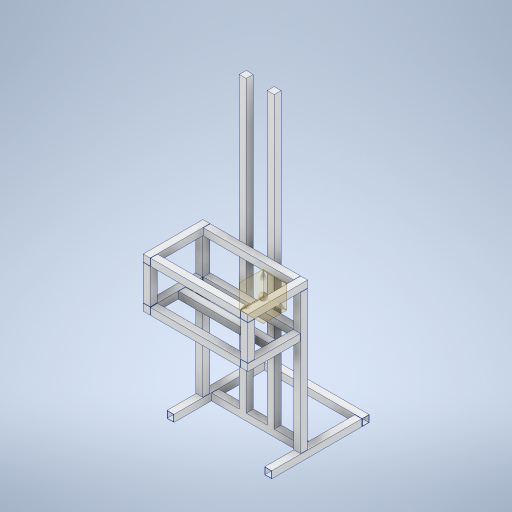
# Autodesk Inventor part: Новый каркас
Saved by Autodesk Inventor 2023 (Build 270158000, 158)
## iProperties
Created: 2022-04-27
Part Number: Новый каркас
Material: Алюминий 6061
Document SubType Name: Modeling
Designer: avkap
Density: 2.7 g/cm^3
Appearance: Алюминий — плоский
Mass: 63771.5 g
Surface Area: 27844 cm^2
Volume: 23619.1 cm^3
Author: avkap
Autodesk Inventor part; units mm, degrees
ref_plane "YZ Plane" through (0, 0, 0) normal (1, 0, 0) x (0, 1, 0)
ref_plane "XZ Plane" through (0, 0, 0) normal (0, 1, 0) x (-1, 0, 0)
ref_plane "XY Plane" through (0, 0, 0) normal (0, 0, 1) x (1, 0, 0)
sketch "Эскиз1" plane through (0, 0, 0) normal (0, 1, 0) x (-1, 0, 0)
  line L0 (-600, 0) -> (-600, -300)
  line L1 (-600, -300) -> (0, -300)
  line L2 (0, -300) -> (0, -42)
  line L3 (-600, 0) -> (-600, -40)
  line L4 (0, -300) -> (0, -260)
  line L5 (0, -260) -> (-600, -260)
  line L6 (-600, -40) -> (-600, -42)
  line L7 (-600, -42) -> (-560, -42)
  line L8 (-560, -42) -> (-560, -208)
  line L9 (0, -42) -> (-40, -42)
  line L10 (-40, -42) -> (-40, -258)
  line L11 (-40, -258) -> (0, -258)
  line L12 (-560, -208) -> (-560, -258)
  line L13 (-560, -258) -> (-600, -258)
  point P0 (0, 0)
  point P1 (-600, -208)
  dimension "d0" = 600
  dimension "d1" = 300
  dimension "d3" = 40
  dimension "d4" = 2
  dimension "d5" = 40
  dimension "d7" = 40
  dimension "d69" = 216
  constraints: 28 end point, 10 point on line, 4 perpendicular, 2 parallel
  measures "d0" distance of L1.end L0.end
  measures "d1" distance of L0.end L0.start
  measures "d3" distance of L1.end L4.end
  measures "d4" distance of L3.end L6.end
  measures "d5" distance of L6.end L7.end
  measures "d7" distance of L2.end L9.end
  measures "d69" distance of L9.end L10.end
ref_plane "РабПлоскость2" through (0, 860, 0) normal (0, 1, 0) x (1, 0, 0)
ref_plane "РабПлоскость6" through (0, 0, 0) normal (0, -1, 0) x (1, 0, 0)
sketch "Эскиз5" plane through (0, 0, 0) normal (0, -1, 0) x (1, 0, 0)
  line L0 (0, 0) -> (40, 0) projected
  line L1 (0, 0) -> (300, 0)
  line L2 (300, 0) -> (300, 2)
  line L3 (300, 2) -> (280, 2)
  line L4 (320, 2) -> (300, 2)
  line L5 (300, 2) -> (200, 2)
  line L6 (200, 2) -> (200, 4)
  line L7 (200, 4) -> (400, 4)
  line L8 (200, 4) -> (240, 4)
  line L9 (240, 4) -> (240, 44)
  line L10 (240, 44) -> (200, 44)
  line L11 (200, 44) -> (200, 4)
  line L12 (400, 4) -> (360, 4)
  line L13 (360, 4) -> (360, 44)
  line L14 (360, 44) -> (400, 44)
  line L15 (400, 44) -> (400, 4)
  dimension "d19" = 300
  dimension "d20" = 2
  dimension "d146" = 100
  dimension "d147" = 2
  dimension "d148" = 200
  dimension "d149" = 40
  dimension "d150" = 40
  dimension "d151" = 40
  dimension "d152" = 40
  constraints: 30 end point, 4 parallel, 4 perpendicular, 2 collinear, 2 horizontal, 2 point on line, 2 vertical
  measures "d19" distance of L0.start L1.end
  measures "d20" distance of L1.end L2.end
  measures "d146" distance of L2.end L5.end
  measures "d147" distance of L5.end L6.end
  measures "d148" distance of L6.end L7.end
  measures "d149" distance of L10.end L9.end
  measures "d150" distance of L9.end L8.end
  measures "d151" distance of L13.end L14.end
  measures "d152" distance of L12.end L13.end
extrude "Выдавливание10" add sketch "Эскиз1" along normal blind 40
extrude "Выдавливание20" add sketch "Эскиз5" against normal blind 1700
ref_plane "РабПлоскость16" through (200, 900, 44) normal (0, 0, 1) x (1, 0, 0)
sketch "Эскиз19" plane through (200, 900, 44) normal (0, 0, 1) x (1, 0, 0)
  line L0 (0, -900) -> (0, 800) projected
  line L1 (0, 800) -> (200, 800)
  line L2 (200, 800) -> (200, 600)
  line L3 (200, 600) -> (0, 600)
  line L4 (0, 600) -> (0, 800)
  line L5 (100, 600) -> (100, 800)
  line L6 (100, 600) -> (100, 700)
  line L7 (100, 700) -> (100, 692.5)
  line L8 (100, 692.5) -> (100, 709.5)
  circle A0 centre (100, 709.5) radius 2
  circle A1 centre (100, 692.5) radius 2
  line L9 (40, 800) -> (0, 800) projected
  line L10 (20, 800) -> (20, 600)
  line L11 (160, 800) -> (200, 800) projected
  line L12 (180, 800) -> (180, 600)
  line L13 (180, 600) -> (180, 620)
  line L14 (180, 620) -> (20, 620)
  line L15 (40, 800) -> (20, 800)
  line L16 (20, 800) -> (20, 780)
  line L17 (20, 780) -> (40, 780)
  line L18 (40, 780) -> (40, 800)
  line L19 (40, 780) -> (200, 780)
  circle A2 centre (20, 780) radius 3
  circle A3 centre (20, 620) radius 3
  circle A4 centre (180, 780) radius 3
  circle A5 centre (180, 620) radius 3
  point P0 (-200, -900)
  dimension "d156" = 200
  dimension "d157" = 200
  dimension "d266" = 100
  dimension "d267" = 7.5
  dimension "d268" = 17
  dimension "d269" = 4
  dimension "d270" = 4
  dimension "d271" = 20
  dimension "d272" = 20
  dimension "d273" = 20
  dimension "d274" = 6
  dimension "d275" = 6
  dimension "d276" = 6
  dimension "d277" = 6
  constraints: 34 end point, 9 point on line, 6 centre point, 5 coincident, 5 midpoint, 4 parallel, 3 horizontal, 3 perpendicular
  measures "d156" distance of L2.end L3.end
  measures "d157" distance of L1.end L2.end
  measures "d266" distance of L5.start L6.end
  measures "d267" distance of L6.end L7.end
  measures "d268" distance of L7.end L8.end
  measures "d269" diameter of A0
  measures "d270" diameter of A1
  measures "d271" distance of L12.end L13.end
  measures "d272" distance of L17.end L16.end
  measures "d273" distance of L16.end L15.end
  measures "d274" diameter of A2
  measures "d275" diameter of A3
  measures "d276" diameter of A4
  measures "d277" diameter of A5
extrude "Выдавливание21" [suppressed]
sketch "Эскиз23" plane through (560, 0, -42) normal (0, 0, 1) x (1, 0, 0)
  line L0 (-520, 0) -> (-520, 40) projected
  line L1 (-520, 0) -> (-560, 0)
  line L2 (-560, 0) -> (-560, 40)
  line L3 (-560, 40) -> (-520, 40)
  line L4 (-520, 40) -> (-520, 0)
  line L5 (40, 0) -> (40, 40) projected
  line L6 (40, 0) -> (0, 0)
  line L7 (0, 0) -> (0, 40)
  line L8 (0, 40) -> (40, 40)
  line L9 (40, 40) -> (40, 0)
  constraints: 16 end point, 4 parallel, 2 horizontal, 2 perpendicular
extrude "Выдавливание25" add sketch "Эскиз23" along normal blind 300
ref_plane "РабПлоскость12" through (42, 0, -258) normal (1, 0, 0) x (0, 0, -1)
sketch "Эскиз26" plane through (42, 0, -258) normal (1, 0, 0) x (0, 0, -1)
  line L0 (-302, 40) -> (-262, 40)
  line L1 (-262, 40) -> (-262, 0)
  line L2 (-262, 0) -> (-302, 0)
  line L3 (-302, 0) -> (-302, 40)
  line L4 (-262, 0) -> (0, 0)
  line L5 (0, 0) -> (0, 40) projected
  line L6 (0, 0) -> (0, 40)
  line L7 (-302, 0) -> (-302, 1700) projected
  point P0 (-258, 0)
  point P1 (-302, 1500)
  dimension "d189" = 40
  dimension "d302" = 262
  constraints: 12 end point, 2 horizontal, 2 parallel, 2 perpendicular
  measures "d189" distance of L1.end L2.end
  measures "d302" distance of L1.end L4.end
extrude "Выдавливание26" add sketch "Эскиз26" along normal blind 516
ref_plane "РабПлоскость22" through (0, 600, 0) normal (0, -1, 0) x (1, 0, 0)
ref_plane "РабПлоскость15" through (0, 42, 0) normal (0, 1, 0) x (1, 0, 0)
sketch "Эскиз30" plane through (0, 42, 0) normal (0, 1, 0) x (1, 0, 0)
  line L0 (40, 258) -> (40, -258) projected
  line L1 (40, -52.0658) -> (0, -52.0658)
  line L2 (0, -52.0658) -> (0, -92.0658)
  line L3 (0, -92.0658) -> (40, -92.0658)
  line L4 (40, -92.0658) -> (40, -52.0658)
  line L5 (560, 258) -> (560, -258) projected
  line L6 (560, -52.0658) -> (600, -52.0658)
  line L7 (600, -52.0658) -> (600, -92.0658)
  line L8 (600, -92.0658) -> (560, -92.0658)
  line L9 (560, -92.0658) -> (560, -52.0658)
  point P0 (0, 0)
  dimension "d217" = 40
  dimension "d218" = 40
  constraints: 16 end point, 4 parallel, 4 point on line, 2 horizontal, 2 perpendicular
  measures "d217" distance of L3.end L2.end
  measures "d218" distance of L2.end L1.end
extrude "Выдавливание28" add sketch "Эскиз30" along normal blind 800
ref_plane "РабПлоскость18" through (0, 844, 0) normal (0, 1, 0) x (1, 0, 0)
ref_plane "РабПлоскость21" through (42, 600, 294) normal (1, 0, 0) x (0, 0, -1)
sketch "Эскиз40" plane through (42, 600, 294) normal (1, 0, 0) x (0, 0, -1)
  line L0 (200, 40) -> (200, 0)
  line L1 (60, 40) -> (100, 40)
  line L2 (100, 40) -> (100, 0)
  line L3 (100, 0) -> (60, 0)
  line L4 (60, 0) -> (60, 40)
  line L5 (100, 0) -> (200, 0)
  line L6 (201.9342, -558) -> (201.9342, 242) projected
  point P0 (294, -600)
  dimension "d297" = 40
  dimension "d298" = 40
  dimension "d326" = 100
  constraints: 12 end point, 2 parallel, 2 perpendicular, 1 horizontal
  measures "d297" distance of L2.end L3.end
  measures "d298" distance of L1.end L2.end
  measures "d326" distance of L2.end L0.end
extrude "Выдавливание36" add sketch "Эскиз40" along normal blind 516
sketch "Эскиз41" plane through (0, 600, 0) normal (0, -1, 0) x (1, 0, 0)
  line L0 (560, 92.0658) -> (600, 92.0658) projected
  line L1 (0, 92.0658) -> (40, 92.0658) projected
  line L2 (600, 92.0658) -> (600, 94.0658)
  line L3 (600, 94.0658) -> (560, 94.0658)
  line L4 (560, 94.0658) -> (560, 394.0658)
  line L5 (560, 394.0658) -> (600, 394.0658)
  line L6 (600, 394.0658) -> (600, 94.0658)
  line L7 (0, 92.0658) -> (40, 92.0658)
  line L8 (0, 92.0658) -> (0, 94.0658)
  line L9 (0, 94.0658) -> (40, 94.0658)
  line L10 (40, 94.0658) -> (40, 394.0658)
  line L11 (40, 394.0658) -> (0, 394.0658)
  line L12 (0, 394.0658) -> (0, 94.0658)
  line L13 (40, 394.0658) -> (42, 394.0658)
  line L14 (42, 394.0658) -> (42, 354.0658)
  line L15 (560, 394.0658) -> (558, 394.0658)
  line L16 (558, 394.0658) -> (558, 354.0658)
  line L17 (558, 354.0658) -> (42, 354.0658)
  line L18 (42, 394.0658) -> (558, 394.0658)
  point P0 (0, 0)
  point P1 (560, 294)
  dimension "d304" = 2
  dimension "d305" = 40
  dimension "d306" = 300
  dimension "d308" = 2
  dimension "d309" = 300
  dimension "d310" = 2
  dimension "d311" = 40
  dimension "d312" = 2
  dimension "d313" = 40
  constraints: 34 end point, 11 perpendicular, 2 point on line, 2 vertical, 1 horizontal
  measures "d304" distance of L0.end L2.end
  measures "d305" distance of L2.end L3.end
  measures "d306" distance of L3.end L4.end
  measures "d308" distance of L1.start L8.end
  measures "d309" distance of L9.end L10.end
  measures "d310" distance of L10.end L13.end
  measures "d311" distance of L13.end L14.end
  measures "d312" distance of L4.end L15.end
  measures "d313" distance of L15.end L16.end
extrude "Выдавливание37" add sketch "Эскиз41" against normal blind 40
ref_plane "РабПлоскость23" through (0, 642, 0) normal (0, 1, 0) x (1, 0, 0)
sketch "Эскиз42" plane through (0, 642, 0) normal (0, 1, 0) x (1, 0, 0)
  line L0 (0, -394.0658) -> (40, -394.0658) projected
  line L1 (0, -394.0658) -> (40, -394.0658)
  line L2 (40, -394.0658) -> (40, -354.0658)
  line L3 (40, -354.0658) -> (0, -354.0658)
  line L4 (0, -354.0658) -> (0, -394.0658)
  line L5 (600, -394.0658) -> (560, -394.0658) projected
  line L6 (560, -394.0658) -> (600, -394.0658)
  line L7 (600, -394.0658) -> (600, -354.0658)
  line L8 (600, -354.0658) -> (560, -354.0658)
  line L9 (560, -354.0658) -> (560, -394.0658)
  point P0 (0, 0)
  dimension "d317" = 40
  dimension "d318" = 40
  dimension "d319" = 40
  dimension "d320" = 40
  constraints: 16 end point, 4 parallel, 2 horizontal, 2 perpendicular
  measures "d317" distance of L3.end L2.end
  measures "d318" distance of L2.end L1.end
  measures "d319" distance of L8.end L7.end
  measures "d320" distance of L7.end L6.end
extrude "Выдавливание38" add sketch "Эскиз42" along normal blind 200
ref_plane "РабПлоскость24" through (42, 42, 92.0658) normal (1, 0, 0) x (0, 0, -1)
sketch "Эскиз43" plane through (42, 42, 92.0658) normal (1, 0, 0) x (0, 0, -1)
  line L0 (-302, 558) -> (-2, 558) projected
  line L1 (-2, 558) -> (40, 558)
  line L2 (40, 0) -> (40, 800) projected
  line L3 (-2, 558) -> (-2, 598) projected
  line L4 (-2, 598) -> (40, 598)
  line L5 (0, 0) -> (0, 800) projected
  line L6 (40, 598) -> (0, 598)
  line L7 (0, 598) -> (0, 558)
  line L8 (0, 558) -> (40, 558)
  line L9 (40, 558) -> (40, 598)
  point P0 (92.0658, -42)
  constraints: 12 end point, 3 horizontal, 3 point on line, 2 parallel, 1 perpendicular
extrude "Выдавливание39" add sketch "Эскиз43" along normal blind 517 contours L5 L4 L2 L1
ref_plane "РабПлоскость25" through (0, 844, 0) normal (0, 1, 0) x (1, 0, 0)
sketch "Эскиз44" plane through (0, 844, 0) normal (0, 1, 0) x (1, 0, 0)
  line L0 (0, -52.0658) -> (0, -92.0658) projected
  line L1 (0, -52.0658) -> (40, -52.0658)
  line L2 (40, -52.0658) -> (40, -394.0658)
  line L3 (40, -394.0658) -> (0, -394.0658)
  line L4 (0, -394.0658) -> (0, -52.0658)
  line L5 (42, -354.0658) -> (42, -394.0658) projected
  line L6 (42, -394.0658) -> (558, -394.0658)
  line L7 (558, -394.0658) -> (558, -354.0658)
  line L8 (558, -354.0658) -> (42, -354.0658)
  line L9 (42, -354.0658) -> (42, -394.0658)
  line L10 (560, -94.0658) -> (560, -394.0658) projected
  line L11 (600, -92.0658) -> (600, -52.0658) projected
  line L12 (560, -394.0658) -> (600, -394.0658)
  line L13 (600, -394.0658) -> (600, -52.0658)
  line L14 (600, -52.0658) -> (560, -52.0658)
  line L15 (560, -52.0658) -> (560, -394.0658)
  line L16 (559, -92.0658) -> (559, -52.0658) projected
  line L17 (559, -52.0658) -> (42, -52.0658)
  line L18 (42, -52.0658) -> (42, -92.0658)
  line L19 (42, -92.0658) -> (559, -92.0658)
  line L20 (559, -92.0658) -> (559, -52.0658)
  point P0 (0, 0)
  dimension "d346" = 40
  dimension "d347" = 342
  constraints: 32 end point, 8 parallel, 4 horizontal, 4 perpendicular, 1 point on line
  measures "d346" distance of L2.end L3.end
  measures "d347" distance of L1.end L2.end
extrude "Выдавливание40" add sketch "Эскиз44" along normal blind 40
sketch "Эскиз45" plane through (560, 0, 258) normal (0, 0, 1) x (1, 0, 0)
  line L0 (-520, 40) -> (-560, 40) projected
  line L1 (-560, 0) -> (-520, 0) projected
  line L2 (-520, 0) -> (-522, 0)
  line L3 (-522, 0) -> (-522, 2)
  line L4 (-560, 40) -> (-558, 40)
  line L5 (-558, 40) -> (-558, 38)
  line L6 (-558, 38) -> (-522, 38)
  line L7 (-522, 38) -> (-522, 2)
  line L8 (-522, 2) -> (-558, 2)
  line L9 (-558, 2) -> (-558, 38)
  line L10 (0, 0) -> (0, 40) projected
  line L11 (0, 40) -> (0, 38)
  line L12 (0, 38) -> (2, 38)
  line L13 (40, 0) -> (40, 2)
  line L14 (40, 0) -> (40, 40) projected
  line L15 (40, 2) -> (38, 2)
  line L16 (38, 2) -> (0, 2)
  line L17 (0, 2) -> (0, 38)
  line L18 (0, 38) -> (38, 38)
  line L19 (38, 38) -> (38, 2)
  line L20 (2, 38) -> (2, 2)
  point P0 (2, 38)
  point P1 (2, 38)
  dimension "d352" = 2
  dimension "d353" = 2
  dimension "d354" = 2
  dimension "d355" = 2
  dimension "d356" = 2
  dimension "d357" = 2
  dimension "d358" = 2
  dimension "d359" = 2
  constraints: 34 end point, 7 perpendicular, 5 point on line, 4 parallel, 2 horizontal
  measures "d352" distance of L1.end L2.end
  measures "d353" distance of L2.end L3.end
  measures "d354" distance of L0.end L4.end
  measures "d355" distance of L4.end L5.end
  measures "d356" distance of L10.end L11.end
  measures "d357" distance of L11.end L12.end
  measures "d358" distance of L13.start L13.end
  measures "d359" distance of L13.end L15.end
extrude "Выдавливание41" cut sketch "Эскиз45" against normal blind 518.75 contours L6 L7 L8 L9 | L20 L18 L19 L16
sketch "Эскиз46" plane through (600, 0, -260) normal (1, 0, 0) x (0, 0, -1)
  line L0 (0, 0) -> (0, 40) projected
  line L1 (0, 40) -> (2, 40)
  line L2 (2, 40) -> (2, 38)
  line L3 (2, 38) -> (0, 38)
  line L4 (0, 38) -> (0, 40)
  line L5 (2, 38) -> (38, 38)
  line L6 (38, 38) -> (38, 2)
  line L7 (38, 2) -> (2, 2)
  line L8 (2, 2) -> (2, 38)
  point P0 (-260, 0)
  dimension "d362" = 2
  dimension "d363" = 2
  dimension "d364" = 36
  dimension "d365" = 36
  constraints: 16 end point, 4 parallel, 2 horizontal, 2 perpendicular
  measures "d362" distance of L2.end L3.end
  measures "d363" distance of L1.end L2.end
  measures "d364" distance of L6.end L7.end
  measures "d365" distance of L5.end L6.end
extrude "Выдавливание42" cut sketch "Эскиз46" against normal blind 929.5 contours L5 L6 L7 L8
